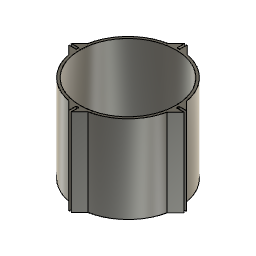
HALEFINNE HOLDER V4 v1 (Autodesk Fusion 360 design; units mm, degrees)
Autodesk Fusion 360 part; units mm, degrees
sketch "Sketch1" plane through (0, 0, 0) normal (0, 0, 1) x (1, 0, 0)
  circle A0 centre (0, 0) radius 38.5
  circle A1 centre (0, 0) radius 40.5
  line L0 (40.497, 0.49) -> (46.497, 0.49)
  line L1 (46.497, 0.49) -> (39.8697, 7.1173)
  line L2 (46.497, 0.49) -> (37.1246, 0.49) construction
  line L3 (46.497, 0.49) -> (46.497, -1.51) construction
  line L4 (37.1246, 0.49) -> (37.1246, -1.51) construction
  line L5 (37.1246, -1.51) -> (40.4718, -1.51) construction
  line L6 (40.4718, -1.51) -> (46.4718, -1.51)
  line L7 (46.4718, -1.51) -> (39.6294, -8.3525)
  line L8 (-1, 37) -> (1, 37) construction
  line L9 (1, 37) -> (1, 40.4877) construction
  line L10 (-1, 37) -> (-1, 40.4877) construction
  line L11 (-1, 40.4877) -> (-1, 46.4877)
  line L12 (-1, 46.4877) -> (-7.7327, 39.7549)
  line L13 (1, 40.4877) -> (1, 46.4877)
  line L14 (1, 46.4877) -> (7.7327, 39.7549)
  line L15 (-35, 1) -> (-35, -1) construction
  line L16 (-35, -1) -> (-40.4877, -1) construction
  line L17 (-35, 1) -> (-40.4877, 1) construction
  line L18 (-40.4877, -1) -> (-46.4877, -1)
  line L19 (-46.4877, -1) -> (-39.7549, -7.7327)
  line L20 (-40.4877, 1) -> (-46.4877, 1)
  line L21 (-46.4877, 1) -> (-39.7549, 7.7327)
  line L22 (-1, -37.5) -> (1, -37.5) construction
  line L23 (1, -37.5) -> (1, -40.4877) construction
  line L24 (-1, -37.5) -> (-1, -40.4877) construction
  line L25 (-1, -40.4877) -> (-1, -46.4877)
  line L26 (-1, -46.4877) -> (-7.7327, -39.7549)
  line L27 (1, -40.4877) -> (1, -46.4877)
  line L28 (1, -46.4877) -> (7.7327, -39.7549)
  dimension "d5" = 77
  dimension "d6" = 81
  dimension "d7" = 81
  dimension "d8" = 6
  dimension "d9" = 45
  dimension "d10" = 2
  dimension "d11" = 2
  dimension "d12" = 6
  dimension "d13" = 45
  dimension "d14" = 2
  dimension "d15" = 6
  dimension "d16" = 45
  dimension "d17" = 6
  dimension "d18" = 45
  dimension "d19" = 2
  dimension "d20" = 6
  dimension "d21" = 45
  dimension "d22" = 6
  dimension "d23" = 45
  dimension "d24" = 2
  dimension "d25" = 6
  dimension "d26" = 45
  dimension "d27" = 6
  dimension "d28" = 45
  constraint coincident A0.centre A1.centre
  constraint coincident A1 L0.start
  constraint horizontal L0
  constraint horizontal L2
  constraint coincident A1 L1.end
  constraint perpendicular L0 L3
  constraint perpendicular L2 L4
  constraint coincident A1 L5.end
  constraint perpendicular L4 L5
  constraint perpendicular L3 L6
  constraint coincident A1 L7.end
  constraint perpendicular L3 L8
  constraint coincident A1 L9.end
  constraint perpendicular L8 L9
  constraint coincident A1 L10.end
  constraint perpendicular L8 L10
  constraint parallel L10 L11
  constraint coincident A1 L12.end
  constraint parallel L9 L13
  constraint coincident A1 L14.end
  constraint parallel L9 L15
  constraint coincident A1 L16.end
  constraint perpendicular L9 L16
  constraint coincident A1 L17.end
  constraint perpendicular L15 L17
  constraint perpendicular L15 L18
  constraint coincident A1 L19.end
  constraint parallel L17 L20
  constraint coincident A1 L21.end
  constraint parallel L17 L22
  constraint coincident A1 L23.end
  constraint perpendicular L22 L23
  constraint coincident A1 L24.end
  constraint perpendicular L22 L24
  constraint parallel L24 L25
  constraint coincident A1 L26.end
  constraint parallel L23 L27
  constraint coincident A1 L28.end
  measures "d5" diameter of A0
  measures "d6" diameter of A1
  measures "d7" diameter of A1
  measures "d8" distance of L0.start L0.end
  measures "d9" angle of L1 L2
  measures "d10" distance of L0.end L3.end
  measures "d11" distance of L2.end L4.end
  measures "d12" distance of L5.end L6.end
  measures "d13" angle of L6 L7
  measures "d14" distance of L8.start L8.end
  measures "d15" distance of L10.end L11.end
  measures "d16" angle of L11 L12
  measures "d17" distance of L9.end L13.end
  measures "d18" angle of L13 L14
  measures "d19" distance of L15.start L15.end
  measures "d20" distance of L16.end L18.end
  measures "d21" angle of L18 L19
  measures "d22" distance of L17.end L20.end
  measures "d23" angle of L20 L21
  measures "d24" distance of L22.start L22.end
  measures "d25" distance of L24.end L25.end
  measures "d26" angle of L25 L26
  measures "d27" distance of L23.end L27.end
  measures "d28" angle of L27 L28
extrude "Extrude1" add sketch "Sketch1" along normal blind 70
equation "ytredim = 77 mm"
equation "lengdeholder = 6 mm"
equation "breddeholder = 2 mm"
equation "gradholder = 45 deg"
equation "d5 = ytredim"
equation "d6 = ytredim + 4 mm"
equation "d8 = lengdeholder"
equation "d9 = gradholder"
equation "d10 = breddeholder"
equation "d11 = breddeholder"
equation "d12 = lengdeholder"
equation "d13 = gradholder"
equation "d14 = breddeholder"
equation "d15 = lengdeholder"
equation "d16 = gradholder"
equation "d17 = lengdeholder"
equation "d18 = gradholder"
equation "d19 = breddeholder"
equation "d20 = lengdeholder"
equation "d21 = gradholder"
equation "d22 = lengdeholder"
equation "d23 = gradholder"
equation "d24 = breddeholder"
equation "d25 = lengdeholder"
equation "d26 = gradholder"
equation "d27 = lengdeholder"
equation "d28 = gradholder"
